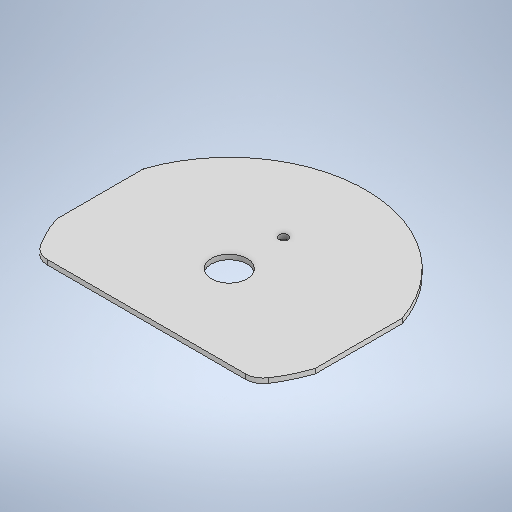
# Autodesk Inventor part: tapa_carcasa_4.0
Saved by Autodesk Inventor 2025.3 (Build 293356030, 356C)
## iProperties
Created: 2025-10-09
Part Number: tapa_carcasa_4.0
Material: Generic
Document SubType Name: Modeling
Designer: brene
Density: 1 g/cm^3
Appearance: Default
Author: brene
Autodesk Inventor part; units mm, degrees
ref_plane "YZ Plane" through (0, 0, 0) normal (1, 0, 0) x (0, 1, 0)
ref_plane "XZ Plane" through (0, 0, 0) normal (0, 1, 0) x (-1, 0, 0)
ref_plane "XY Plane" through (0, 0, 0) normal (0, 0, 1) x (1, 0, 0)
sketch "Sketch3" plane through (0, 0, 0) normal (0, 1, 0) x (-1, 0, 0)
  line L0 (0, 0) -> (72.5, 0)
  line L1 (0, 0) -> (0, 46.5)
  line L2 (72.5, 24.4131) -> (72.5, -24.4131)
  line L3 (0, 46.5) -> (55.5878, 46.5)
  line L4 (-72.5, 24.4131) -> (-72.5, -24.4131)
  line L5 (0, 46.5) -> (-55.5878, 46.5)
  arc A0 (72.5, 24.4131) -> (63.9468, 41.9887) centre (0, 0) ccw
  arc A1 (-63.9468, 41.9887) -> (-72.5, 24.4131) centre (0, 0) ccw
  arc A2 (-72.5, -24.4131) -> (72.5, -24.4131) centre (0, 0) ccw
  arc A3 (63.9468, 41.9887) -> (55.5878, 46.5) centre (55.5878, 36.5) ccw
  arc A4 (-55.5878, 46.5) -> (-63.9468, 41.9887) centre (-55.5878, 36.5) ccw
  point P0 (60.7454, 46.5)
  point P1 (-60.7454, 46.5)
  dimension "d28" = 72.5
  dimension "d29" = 46.5
  dimension "d30" = 10
  dimension "d31" = 10
  dimension "d32" = 76.5
  dimension "d34" = 72.5
  dimension "d35" = 76.5
  constraints: 12 end point, 12 point on circle, 5 centre point, 4 tangent, 3 symmetric about line, 2 horizontal, 2 point on line, 1 perpendicular, 1 vertical
  measures "d28" distance of L0.start L0.end
  measures "d29" distance of L0.start L1.end
  measures "d30" radius of A3
  measures "d31" radius of A4
  measures "d32" radius of A2
  measures "d34" distance between parallel lines of L2 L1
  measures "d35" radius of A1
extrude "Extrusion2" add sketch "Sketch3" along normal blind 2.7
sketch "Sketch4" plane through (0, 2.7, 0) normal (0, 1, 0) x (1, 0, 0)
  line L0 (-55.5878, -46.5) -> (55.5878, -46.5) projected
  line L1 (0, -46.5) -> (0, 0)
  circle A0 centre (0, 0) radius 10
  arc A1 (72.5, 24.4131) -> (-72.5, 24.4131) centre (0, 0) ccw projected
  line L2 (0, 76.5) -> (0, 30.5)
  circle A2 centre (0, 30.5) radius 2.5
  dimension "d36" = 20
  dimension "d37" = 46
  dimension "d38" = 5
  constraints: 4 end point, 2 centre point, 2 coincident, 2 vertical, 1 midpoint, 1 point on circle
  measures "d36" diameter of A0
  measures "d37" distance of L2.start L2.end
  measures "d38" diameter of A2
extrude "Extrusion3" cut sketch "Sketch4" against normal blind 10
body "Solid2"
